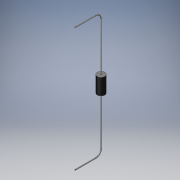
# Autodesk Inventor part: Diode
Saved by Autodesk Inventor 2019 (Build 230136000, 136)
## iProperties
Created: 2020-03-29
Part Number: Diode
Material: Silicon Nitride
Document SubType Name: Modeling
Designer: darkl
Density: 3.18 g/cm^3
Appearance: Anodized - Light Gray
Author: darkl
Autodesk Inventor part; units mm, degrees
ref_plane "YZ Plane" through (0, 0, 0) normal (1, 0, 0) x (0, 1, 0)
ref_plane "XZ Plane" through (0, 0, 0) normal (0, 1, 0) x (-1, 0, 0)
ref_plane "XY Plane" through (0, 0, 0) normal (0, 0, 1) x (1, 0, 0)
sketch "Sketch1" plane through (0, 0, 0) normal (0, 1, 0) x (-1, 0, 0)
  point P0 (0, 0)
sketch "Sketch2" plane through (0, 0, 0) normal (0, 1, 0) x (-1, 0, 0)
  circle A0 centre (0.2711, 0.2358) radius 1.75
  point P0 (0, 0)
  dimension "d0" = 3.5
  constraints: 1 centre point
  measures "d0" diameter of A0
extrude "Extrusion1" add sketch "Sketch2" along normal blind 7.5
sketch "Sketch5" plane through (-0.2711, 7.5, 0.2358) normal (0, 1, 0) x (1, 0, 0)
  circle A0 centre (0, 0) radius 0.25 projected
  point P0 (0.2711, 0.2358)
sketch "Sketch8" plane through (-0.2711, 0, 0.2358) normal (0, -1, 0) x (1, 0, 0)
  circle A0 centre (0, 0) radius 0.25
  point P0 (0.2711, -0.2358)
  dimension "d24" = 0.5
  constraints: 1 centre point
  measures "d24" diameter of A0
sketch3d "3D Sketch3"
  line L0 (-0.2711, 0, 0.2358) -> (-0.2711, -22.5, 0.2358)
  arc A0 (-0.2711, -22.5, 0.2358) -> (-0.2711, -25, 2.7358) centre (-0.2711, -22.5, 2.7358) ccw
  line L1 (-0.2711, -25, 2.7358) -> (-0.2711, -25, 12.2358)
  dimension "d21" = 25
  dimension "d22" = 12
  dimension "d23" = 2.5
sweep "Sweep1" add profiles "Sketch8" path "3D Sketch3"
sketch3d "3D Sketch5"
  line L0 (-0.2711, 7.5, 0.2358) -> (-0.2711, 30, 0.2358)
  arc A0 (-0.2711, 30, 0.2358) -> (-0.2711, 32.5, 2.7358) centre (-0.2711, 30, 2.7358) ccw
  line L1 (-0.2711, 32.5, 2.7358) -> (-0.2711, 32.5, 12.2358)
  dimension "d27" = 25
  dimension "d28" = 12
  dimension "d29" = 2.5
sweep "Sweep2" add profiles "Sketch5" path "3D Sketch5"
body "Solid1"
